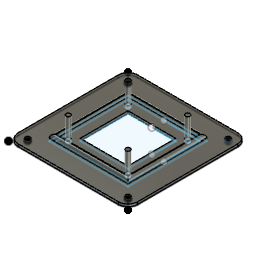
Schalter Halterplatte (Autodesk Fusion 360 design; units mm, degrees)
Autodesk Fusion 360 part; units mm, degrees
sketch "Skizze1" plane through (0, 0, 0) normal (0, 0, 1) x (1, 0, 0)
  line L0 (8, 0) -> (92, 0)
  line L1 (100, 8) -> (100, 92)
  line L2 (92, 100) -> (8, 100)
  line L3 (0, 92) -> (0, 8)
  arc A0 (8, 100) -> (0, 92) centre (8, 92) ccw
  arc A1 (100, 92) -> (92, 100) centre (92, 92) ccw
  arc A2 (92, 0) -> (100, 8) centre (92, 8) ccw
  arc A3 (0, 8) -> (8, 0) centre (8, 8) ccw
  circle A4 centre (8, 8) radius 2
  circle A5 centre (92, 8) radius 2
  circle A6 centre (92, 92) radius 2
  circle A7 centre (8, 92) radius 2
  line L4 (70, 50) -> (70, 70)
  line L5 (70, 70) -> (50, 70)
  line L6 (70, 70) -> (30, 70)
  line L7 (30, 70) -> (30, 30)
  line L8 (30, 30) -> (70, 30)
  line L9 (70, 30) -> (70, 70)
  line L10 (0, 100) -> (9.4142, 90.5858)
  line L11 (90.5858, 9.4142) -> (100, 0)
  circle A8 centre (25, 75) radius 1.9
  circle A9 centre (75, 75) radius 1.9
  circle A10 centre (75, 25) radius 1.9
  circle A11 centre (25, 25) radius 1.9
  line L12 (80, 50) -> (80, 80)
  line L13 (80, 80) -> (50, 80)
  line L14 (80, 80) -> (20, 80)
  line L15 (20, 80) -> (20, 20)
  line L16 (20, 20) -> (80, 20)
  line L17 (80, 20) -> (80, 80)
  line L18 (17, 83) -> (83, 83)
  line L19 (83, 83) -> (83, 17)
  line L20 (83, 17) -> (17, 17)
  line L21 (17, 17) -> (17, 83)
  point P0 (100, 0)
  point P1 (0, 100)
  dimension "d1" = 100
  dimension "d2" = 100
  dimension "d3" = 8
  dimension "d4" = 4
  dimension "d5" = 4
  dimension "d6" = 4
  dimension "d9" = 40
  dimension "d10" = 40
  dimension "d11" = 3.8
  dimension "d12" = 3.8
  dimension "d13" = 3.8
  dimension "d14" = 3.8
  constraint horizontal L0
  constraint vertical L1
  constraint horizontal L2
  constraint vertical L3
  constraint coincident P1 L2
  constraint coincident P1 L3
  constraint tangent L2 A0
  constraint tangent L3 A0
  constraint tangent L1 A1
  constraint tangent L2 A1
  constraint equal A0 A1
  constraint coincident P0 L0
  constraint coincident P0 L1
  constraint tangent L0 A2
  constraint tangent L1 A2
  constraint equal A0 A2
  constraint coincident origin L0
  constraint coincident origin L3
  constraint tangent L0 A3
  constraint tangent L3 A3
  constraint equal A0 A3
  constraint concentric A3 A4
  constraint concentric A2 A5
  constraint concentric A1 A6
  constraint concentric A0 A7
  constraint coincident P1 L10.start
  constraint coincident P0 L11.end
  constraint vertical L4
  constraint horizontal L5
  constraint horizontal L6
  constraint vertical L7
  constraint horizontal L8
  constraint vertical L9
  constraint collinear L10 L11
  constraint coincident A7 L10.end
  constraint coincident A5 L11.start
  constraint vertical L12
  constraint horizontal L13
  constraint horizontal L14
  constraint vertical L15
  constraint horizontal L16
  constraint vertical L17
  constraint horizontal L18
  constraint vertical L19
  constraint horizontal L20
  constraint vertical L21
  measures "d1" distance of origin P0
  measures "d2" distance of origin L10.start
  measures "d3" radius of A0
  measures "d4" diameter of A4
  measures "d5" diameter of A5
  measures "d6" diameter of A7
  measures "d9" distance of L4.end L6.end
  measures "d10" distance of L4.end L8.end
  measures "d11" diameter of A8
  measures "d12" diameter of A9
  measures "d13" diameter of A10
  measures "d14" diameter of A11
extrude "Extrusion1" add sketch "Skizze1" along normal blind 2 contours L0 L1 L2 L3 A0 A1 A2 A3
extrude "Extrusion2" add sketch "Skizze1" along normal blind 5 contours L18 L19 L20 L21
extrude "Extrusion3" add sketch "Skizze1" along normal blind 2 contours L12 L13 L14 L15 L16 L17
extrude "Extrusion4" add sketch "Skizze1" along normal blind 19 contours A8 | A9 | A10 | A11
fillet "Abrundung1" radius 2.5 4 edges at (50, 17, 5) (17, 50, 5) (50, 83, 5) (83, 50, 5)
